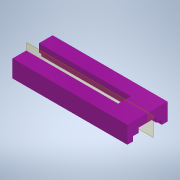
# Autodesk Inventor part: pistonHousingV03-8-in
Saved by Autodesk Inventor 2020.2 (Build 242310000, 310)
## iProperties
Created: 2020-01-19
Part Number: pistonHousingV03-8-in
Material: PET Plastic
Document SubType Name: Modeling
Designer: robst
Density: 1.541 g/cm^3
Appearance: Smooth - Purple
Author: robst
Autodesk Inventor part; units mm, degrees
ref_plane "YZ Plane" through (0, 0, 0) normal (1, 0, 0) x (0, 1, 0)
ref_plane "XZ Plane" through (0, 0, 0) normal (0, 1, 0) x (-1, 0, 0)
sketch "Sketch1" plane through (0, 0, 0) normal (0, 1, 0) x (-1, 0, 0)
  line L0 (127, 44.45) -> (-127, 44.45)
  line L1 (-127, 44.45) -> (-127, -44.45)
  line L2 (-127, -44.45) -> (127, -44.45)
  line L3 (127, -44.45) -> (127, 44.45)
  line L4 (127, 44.45) -> (-127, -44.45) construction
  line L5 (-127, 44.45) -> (127, -44.45) construction
  point P0 (0, 0)
  dimension "d0" = 254
  dimension "d1" = 88.9
  constraints: 12 end point, 2 midpoint, 2 parallel, 1 horizontal, 1 perpendicular
  measures "d0" distance of L0.start L0.end
  measures "d1" distance of L1.end L0.end
extrude "Extrusion1" add sketch "Sketch1" along normal blind 38.1
sketch "Sketch2" plane through (0, 0, 0) normal (0, -1, 0) x (1, 0, 0)
  line L0 (-131.2333, 19.685) -> (-131.2333, -19.685)
  line L1 (-131.2333, -19.685) -> (131.2333, -19.685)
  line L2 (131.2333, -19.685) -> (131.2333, 19.685)
  line L3 (131.2333, 19.685) -> (-131.2333, 19.685)
  line L4 (-131.2333, 19.685) -> (131.2333, -19.685) construction
  line L5 (-131.2333, -19.685) -> (131.2333, 19.685) construction
  point P0 (0, 0)
  dimension "d4" = 39.37
  constraints: 12 end point, 2 midpoint, 2 parallel, 1 perpendicular, 1 vertical
  measures "d4" distance of L0.start L0.end
extrude "Extrusion2" cut sketch "Sketch2" against normal blind 20.32
sketch "Sketch3" plane through (0, 20.32, 0) normal (0, -1, 0) x (1, 0, 0)
  line L0 (-127, -19.685) -> (-127, 19.685) projected
  line L1 (76.2, 13.97) -> (76.2, -13.97)
  line L2 (76.2, -13.97) -> (-127, -13.97)
  line L3 (-127, -13.97) -> (-127, 13.97)
  line L4 (-127, 13.97) -> (76.2, 13.97)
  line L5 (76.2, 13.97) -> (-127, -13.97) construction
  line L6 (76.2, -13.97) -> (-127, 13.97) construction
  point P0 (0, 0)
  point P1 (-25.4, 0)
  point P2 (-127, -13.97)
  dimension "d7" = 101.6
  dimension "d8" = 27.94
  constraints: 12 end point, 2 midpoint, 2 parallel, 1 perpendicular, 1 vertical
  measures "d7" distance from line of point (-25.4, 0) L0
  measures "d8" distance of L1.start L1.end
extrude "Extrusion3" cut sketch "Sketch3" against normal through all
sketch "Sketch4" plane through (0, 0, 0) normal (0, -1, 0) x (1, 0, 0)
  line L0 (127, 31.75) -> (-127, 31.75)
  line L1 (-127, 31.75) -> (-127, -31.75)
  line L2 (-127, -31.75) -> (127, -31.75)
  line L3 (127, -31.75) -> (127, 31.75)
  line L4 (127, 31.75) -> (-127, -31.75) construction
  line L5 (-127, 31.75) -> (127, -31.75) construction
  point P0 (0, 0)
  dimension "d11" = 63.5
  dimension "d12" = 254
  constraints: 12 end point, 2 midpoint, 2 parallel, 1 horizontal, 1 perpendicular
  measures "d11" distance of L1.end L0.end
  measures "d12" distance between parallel lines of L1 L3
extrude "Extrusion4" cut sketch "Sketch4" against normal blind 11.43
sketch "Sketch5" plane through (0, 38.1, 0) normal (0, 1, 0) x (1, 0, 0)
  line L0 (127, 44.45) -> (-127, 44.45) projected
  line L1 (-127, 44.45) -> (-127, 13.97) projected
  line L2 (-101.6, 38.1) -> (127, 38.1) construction
  line L3 (-101.6, 38.1) -> (-101.6, -44.45) construction
  line L4 (-127, -44.45) -> (127, -44.45) construction
  point P0 (0, 0)
  point P1 (-76.2, 38.1)
  point P2 (-50.8, 38.1)
  point P3 (-25.4, 38.1)
  point P4 (0, 38.1)
  point P5 (25.4, 38.1)
  point P6 (50.8, 38.1)
  point P7 (76.2, 38.1)
  point P8 (101.6, 38.1)
  point P9 (-101.6, -38.1)
  point P10 (-76.2, -38.1)
  point P11 (-50.8, -38.1)
  point P12 (-25.4, -38.1)
  point P13 (0, -38.1)
  point P14 (25.4, -38.1)
  point P15 (50.8, -38.1)
  point P16 (76.2, -38.1)
  point P17 (101.6, -38.1)
  dimension "d15" = 6.35
  dimension "d16" = 25.4
  dimension "d19" = 25.4
  dimension "d22" = 76.2
  constraints: 4 end point, 2 horizontal, 2 vertical, 1 point on line, 17 other
  measures "d15" distance from line of L0 L2.start
  measures "d16" distance from line of L2.start L1
  measures "d19" distance of L2.start point (-76.2, 38.1)
  measures "d22" distance of L2.start point (-101.6, -38.1)
hole "Hole1" at (-101.6, 38.1, -38.1) at (-76.2, 38.1, -38.1) at (-50.8, 38.1, -38.1) at (-25.4, 38.1, -38.1) at (0, 38.1, -38.1) at (25.4, 38.1, -38.1) at (50.8, 38.1, -38.1) at (76.2, 38.1, -38.1) at (101.6, 38.1, -38.1) at (-101.6, 38.1, 38.1) at (-76.2, 38.1, 38.1) at (-50.8, 38.1, 38.1) at (-25.4, 38.1, 38.1) at (0, 38.1, 38.1) at (25.4, 38.1, 38.1) at (50.8, 38.1, 38.1) at (76.2, 38.1, 38.1) at (101.6, 38.1, 38.1) direction (0, -1, 0) diameter 5.1054 end through all clearance for "Hex Machine Screw" size "#10" standard "Ansi Unified Screw Threads"
body "Solid1"
